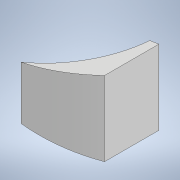
# Autodesk Inventor part: canister holder
Saved by Autodesk Inventor 2021 (Build 250183000, 183)
## iProperties
Created: 2021-08-25
Part Number: canister holder
Material: Generic
Document SubType Name: Modeling
Designer: newic
Density: 1 g/cm^3
Appearance: Default
Author: newic
Autodesk Inventor part; units mm, degrees
ref_plane "YZ Plane" through (0, 0, 0) normal (1, 0, 0) x (0, 1, 0)
ref_plane "XZ Plane" through (0, 0, 0) normal (0, 1, 0) x (-1, 0, 0)
ref_plane "XY Plane" through (0, 0, 0) normal (0, 0, 1) x (1, 0, 0)
sketch "Sketch1" plane through (0, 0, 0) normal (0, 1, 0) x (-1, 0, 0)
  circle A0 centre (0, 0) radius 38.1
  line L0 (-38.1, 0) -> (-41.8338, 0)
  line L1 (-41.8338, 0) -> (-41.8338, 38.1)
  line L2 (-41.8338, 0) -> (-41.8338, -38.1)
  line L3 (-41.8338, -38.1) -> (0, -38.1)
  line L4 (0, 38.1) -> (-41.8338, 38.1)
  arc A1 (0, 38.1) -> (-38.1, 0) centre (0, 0) ccw
  arc A2 (0, 38.1) -> (-26.9408, 26.9408) centre (0, 0) ccw
  arc A3 (-38.1, 0) -> (0, -38.1) centre (0, 0) ccw
  arc A4 (-26.9408, -26.9408) -> (0, -38.1) centre (0, 0) ccw
  arc A5 (-14.5802, 35.1998) -> (-41.8338, 26.9408) centre (-12.1551, -21.8987) ccw
  arc A6 (-41.8338, -26.9408) -> (-14.5802, -35.1998) centre (-12.1551, 21.8987) ccw
  point P0 (-14.5802, -35.1998)
  dimension "d0" = 76.2
  dimension "d1" = 3.7338
  dimension "d2" = 57.15
  dimension "d3" = 57.15
  constraints: 19 point on circle, 10 end point, 7 centre point, 4 tangent, 3 concentric, 2 point on line, 1 coincident, 1 horizontal, 1 parallel, 1 perpendicular, 1 vertical
  measures "d0" diameter of A0
  measures "d1" distance of L0.start L0.end
  measures "d2" radius of A5
  measures "d3" radius of A6
extrude "Extrusion1" add sketch "Sketch1" against normal blind 31.75 contours A0 L0 L1 A5 | A6 L2 L0 A0
sketch "Sketch2" plane through (0, 0, 0) normal (0, 0, 1) x (1, 0, 0)
  line L0 (41.8338, -31.75) -> (-0.6683, -31.75)
  line L1 (41.8338, 0) -> (-9.3567, 0)
  line L2 (41.8338, 0) -> (-14.1234, -9.364)
  line L3 (41.8338, -31.75) -> (-10.3427, -23.0187)
  line L4 (7.8357, -38.2769) -> (6.8485, 14.5363)
  point P0 (0, 0)
  point P1 (7.1202, 0)
  point P2 (7.2285, -5.7909)
  point P3 (7.6066, -26.0223)
  point P4 (7.7137, -31.75)
  dimension "d6" = 9.5
  dimension "d7" = 9.5
  constraints: 10 end point, 2 horizontal
  measures "d6" angle of L3 L0
  measures "d7" angle of L2 L1
extrude "Extrusion2" cut sketch "Sketch2" against normal mid plane 254
sketch "Sketch3" plane through (41.8338, 0, 26.9408) normal (-0.1650476, 0.9862856, 0) x (0.9862856, 0.1650476, 0)
  line L0 (-41.2601, 26.9408) -> (21.7895, 26.9408)
  line L1 (-41.2601, 30.7508) -> (21.7895, 30.7508)
  line L2 (-41.2601, 23.1308) -> (21.7895, 23.1308)
  line L3 (-30.0472, 14.0735) -> (-34.0912, 44.1278)
  line L4 (7.7274, 20.7829) -> (8.5546, 35.8559)
  line L5 (8.5546, 35.8559) -> (-7.3209, 76.3259)
  line L6 (-7.3209, 76.3259) -> (-43.5366, 68.5033)
  line L7 (-43.5366, 68.5033) -> (-33.4602, 39.4386)
  point P0 (7.8563, 23.1308)
  point P1 (-31.2659, 23.1308)
  dimension "d10" = 3.81
  dimension "d11" = 3.81
  constraints: 16 end point, 2 parallel, 1 horizontal, 1 point on line
  measures "d10" distance between parallel lines of L0 L1
  measures "d11" distance between parallel lines of L0 L2
extrude "Extrusion3" cut sketch "Sketch3" against normal blind 254
body "Solid1"
